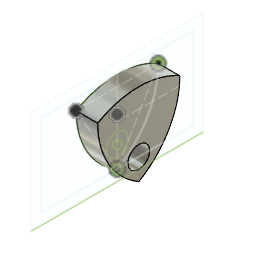
final_oarecum (Autodesk Fusion 360 archive; units mm, degrees)
design "ruleaux"
part number: 2026-06-01-21-01-21-214
Autodesk Fusion 360 part; units mm, degrees
sketch "Excentric Triunghiular Ruleaux + Frame-ul cadrului culisant" plane through (0, 0, 0) normal (1, 0, 0) x (0, 1, 0)
  line L0 (-9.5, 5.4848) -> (0, -10.9697) construction
  line L1 (0, -10.9697) -> (9.5, 5.4848) construction
  line L2 (9.5, 5.4848) -> (-9.5, 5.4848) construction
  arc A0 (0, -10.9697) -> (9.5, 5.4848) centre (-9.5, 5.4848) ccw
  arc A1 (-9.5, 5.4848) -> (0, -10.9697) centre (9.5, 5.4848) ccw
  arc A2 (9.5, 5.4848) -> (-9.5, 5.4848) centre (0, -10.9697) ccw
  circle A3 centre (0, -6) radius 2.5
  line L3 (-17.5, 8.0303) -> (17.5, 8.0303)
  line L4 (17.5, 8.0303) -> (17.5, -10.9697)
  line L5 (17.5, -10.9697) -> (-17.5, -10.9697)
  line L6 (-17.5, -10.9697) -> (-17.5, 8.0303)
  line L7 (0, 8.0303) -> (0, -10.9697) construction
  line L8 (20, -13.4697) -> (-20, -13.4697)
  line L9 (-20, -13.4697) -> (-20, 10.5303)
  line L10 (-20, 10.5303) -> (20, 10.5303)
  line L11 (20, 10.5303) -> (20, -13.4697)
  line L12 (17.5, -1.4697) -> (0, -1.4697) construction
  dimension "d4" = 19
  dimension "d5" = 5
  dimension "d6" = 35
  dimension "d7" = 19
  dimension "d8" = 6
  dimension "d9" = 17.5
  dimension "d10" = -2.5
  constraint coincident L0.start L2.end
  constraint coincident L0.end L1.start
  constraint coincident L0.start A2
  constraint coincident L1.end L2.start
  constraint coincident L0.end A1
  constraint horizontal L3
  constraint vertical L4
  constraint horizontal L5
  constraint vertical L6
  constraint midpoint A2 L7.start
  constraint perpendicular L5 L7
  constraint midpoint L4 L12.start
  constraint midpoint L7 L12.end
  measures "d4" distance of L0.start L1.end
  measures "d5" diameter of A3
  measures "d6" distance of L3.start L3.end
  measures "d7" distance of L3.start L5.end
  measures "d8" distance of origin A3.centre
  measures "d9" distance of L4 L7
extrude "Extrude1" add sketch "Excentric Triunghiular Ruleaux + Frame-ul cadrului culisant" along normal blind 5 contours A0 A1 A2
equation "d9 = ( 35 / 2 ) * 1 mm"
equation "d17 = ( 38 / 2 ) * 1 mm"
named bodies: "Excentric Triunghiular Ruleaux"

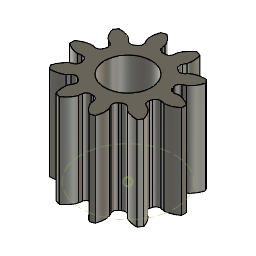
design "gear mic"
part number: 2026-06-01-17-47-26-334
Autodesk Fusion 360 part; units mm, degrees
sketch "Base Circle" plane through (0, 0, 0) normal (0, 0, 1) x (1, 0, 0)
  circle A0 centre (0, 0) radius 3.843
  circle A1 centre (0, 0) radius 2.5
extrude "Extrude3" add sketch "Base Circle" along normal blind 10
sketch "Gear Tooth" plane through (0, 0, 0) normal (0, 0, 1) x (1, 0, 0)
  spline S0 degree 5 poles (4.6331, -0.7809) (4.6369, -0.7816) (4.6445, -0.7827) (4.6559, -0.784) (4.6712, -0.7851) (4.6904, -0.7854) (4.7097, -0.7849) (4.7291, -0.784) (4.7485, -0.7829) (4.7679, -0.7816) (4.7874, -0.7801) (4.8069, -0.7783) (4.8264, -0.7763) (4.8459, -0.7739) (4.8655, -0.7711) (4.8851, -0.768) (4.9048, -0.7646) (4.9244, -0.761) (4.9441, -0.7571) (4.9637, -0.753) (4.9834, -0.7488) (5.0031, -0.7443) (5.0228, -0.7395) (5.0425, -0.7346) (5.0622, -0.7294) (5.0819, -0.7239) (5.1017, -0.7183) (5.1214, -0.7124) (5.1411, -0.7064) (5.1608, -0.7001) (5.1806, -0.6937) (5.2003, -0.6871) (5.22, -0.6802) (5.2397, -0.6732) (5.2594, -0.666) (5.2791, -0.6586) (5.2988, -0.651) (5.3185, -0.6432) (5.3381, -0.6352) (5.3578, -0.6271) (5.3774, -0.6187) (5.3971, -0.6102) (5.4167, -0.6015) (5.4363, -0.5927) (5.4559, -0.5836) (5.4754, -0.5744) (5.495, -0.565) (5.5145, -0.5555) (5.534, -0.5457) (5.5535, -0.5359) (5.573, -0.5258) (5.5924, -0.5156) (5.6119, -0.5052) (5.6313, -0.4946) (5.6506, -0.4839) (5.67, -0.473) (5.6893, -0.4619) (5.7086, -0.4507) (5.7279, -0.4394) (5.7471, -0.4278) (5.7663, -0.4161) (5.7855, -0.4043) (5.8047, -0.3923) (5.8238, -0.3801) (5.8428, -0.3678) (5.8619, -0.3554) (5.8809, -0.3427) (5.8999, -0.33) (5.9188, -0.317) (5.9377, -0.304) (5.9566, -0.2907) (5.9717, -0.28) (5.9829, -0.2719) (5.9904, -0.2665) (5.9942, -0.2638) knots 0 0 0 0 0 0 0.01428571 0.02857143 0.04285714 0.05714286 0.07142857 0.08571429 0.1 0.11428571 0.12857143 0.14285714 0.15714286 0.17142857 0.18571429 0.2 0.21428571 0.22857143 0.24285714 0.25714286 0.27142857 0.28571429 0.3 0.31428571 0.32857143 0.34285714 0.35714286 0.37142857 0.38571429 0.4 0.41428571 0.42857143 0.44285714 0.45714286 0.47142857 0.48571429 0.5 0.51428571 0.52857143 0.54285714 0.55714286 0.57142857 0.58571429 0.6 0.61428571 0.62857143 0.64285714 0.65714286 0.67142857 0.68571429 0.7 0.71428571 0.72857143 0.74285714 0.75714286 0.77142857 0.78571429 0.8 0.81428571 0.82857143 0.84285714 0.85714286 0.87142857 0.88571429 0.9 0.91428571 0.92857143 0.94285714 0.95714286 0.97142857 0.98571429 1 1 1 1 1 1
  spline S1 degree 5 poles (4.6331, 0.7809) (4.6369, 0.7816) (4.6445, 0.7827) (4.6559, 0.784) (4.6712, 0.7851) (4.6904, 0.7854) (4.7097, 0.7849) (4.7291, 0.784) (4.7485, 0.7829) (4.7679, 0.7816) (4.7874, 0.7801) (4.8069, 0.7783) (4.8264, 0.7763) (4.8459, 0.7739) (4.8655, 0.7711) (4.8851, 0.768) (4.9048, 0.7646) (4.9244, 0.761) (4.9441, 0.7571) (4.9637, 0.753) (4.9834, 0.7488) (5.0031, 0.7443) (5.0228, 0.7395) (5.0425, 0.7346) (5.0622, 0.7294) (5.0819, 0.7239) (5.1017, 0.7183) (5.1214, 0.7124) (5.1411, 0.7064) (5.1608, 0.7001) (5.1806, 0.6937) (5.2003, 0.6871) (5.22, 0.6802) (5.2397, 0.6732) (5.2594, 0.666) (5.2791, 0.6586) (5.2988, 0.651) (5.3185, 0.6432) (5.3381, 0.6352) (5.3578, 0.6271) (5.3774, 0.6187) (5.3971, 0.6102) (5.4167, 0.6015) (5.4363, 0.5927) (5.4559, 0.5836) (5.4754, 0.5744) (5.495, 0.565) (5.5145, 0.5555) (5.534, 0.5457) (5.5535, 0.5359) (5.573, 0.5258) (5.5924, 0.5156) (5.6119, 0.5052) (5.6313, 0.4946) (5.6506, 0.4839) (5.67, 0.473) (5.6893, 0.4619) (5.7086, 0.4507) (5.7279, 0.4394) (5.7471, 0.4278) (5.7663, 0.4161) (5.7855, 0.4043) (5.8047, 0.3923) (5.8238, 0.3801) (5.8428, 0.3678) (5.8619, 0.3554) (5.8809, 0.3427) (5.8999, 0.33) (5.9188, 0.317) (5.9377, 0.304) (5.9566, 0.2907) (5.9717, 0.28) (5.9829, 0.2719) (5.9904, 0.2665) (5.9942, 0.2638) knots 0 0 0 0 0 0 0.01428571 0.02857143 0.04285714 0.05714286 0.07142857 0.08571429 0.1 0.11428571 0.12857143 0.14285714 0.15714286 0.17142857 0.18571429 0.2 0.21428571 0.22857143 0.24285714 0.25714286 0.27142857 0.28571429 0.3 0.31428571 0.32857143 0.34285714 0.35714286 0.37142857 0.38571429 0.4 0.41428571 0.42857143 0.44285714 0.45714286 0.47142857 0.48571429 0.5 0.51428571 0.52857143 0.54285714 0.55714286 0.57142857 0.58571429 0.6 0.61428571 0.62857143 0.64285714 0.65714286 0.67142857 0.68571429 0.7 0.71428571 0.72857143 0.74285714 0.75714286 0.77142857 0.78571429 0.8 0.81428571 0.82857143 0.84285714 0.85714286 0.87142857 0.88571429 0.9 0.91428571 0.92857143 0.94285714 0.95714286 0.97142857 0.98571429 1 1 1 1 1 1
  arc A0 (5.9942, -0.2638) -> (5.9942, 0.2638) centre (0, 0) ccw
  line L0 (3.7797, -0.6371) -> (4.6331, -0.7809)
  line L1 (3.7797, 0.6371) -> (4.6331, 0.7809)
  line L2 (3.7797, -0.6371) -> (3.7797, 0.6371)
  point P0 (4.7268, -0.7841)
  point P1 (4.8223, -0.7767)
  point P2 (4.9187, -0.762)
  point P3 (5.0159, -0.7412)
  point P4 (5.1136, -0.7147)
  point P5 (5.2117, -0.6831)
  point P6 (5.31, -0.6465)
  point P7 (5.4084, -0.6052)
  point P8 (5.5068, -0.5592)
  point P9 (5.6051, -0.5088)
  point P10 (5.7031, -0.4539)
  point P11 (5.8006, -0.3948)
  point P12 (5.8977, -0.3314)
  point P13 (4.7268, 0.7841)
  point P14 (4.8223, 0.7767)
  point P15 (4.9187, 0.762)
  point P16 (5.0159, 0.7412)
  point P17 (5.1136, 0.7147)
  point P18 (5.2117, 0.6831)
  point P19 (5.31, 0.6465)
  point P20 (5.4084, 0.6052)
  point P21 (5.5068, 0.5592)
  point P22 (5.6051, 0.5088)
  point P23 (5.7031, 0.4539)
  point P24 (5.8006, 0.3948)
  point P25 (5.8977, 0.3314)
extrude "Extrude4" add sketch "Gear Tooth" along normal blind 10
fillet "Fillet2" radius 0.5 2 edges at (3.7895, -0.6387, 5) (3.7895, 0.6387, 5)
pattern_circular "C-Pattern2" count 10 over 360 about axis through (0, 0, 0) along (0, 0, 1) of "Extrude4", "Fillet2"
sketch "Diametrial Pitch Circle" plane through (0, 0, 0) normal (0, 0, 1) x (1, 0, 0)
  circle A0 centre (0, 0) radius 5 construction
named bodies: "Spur Gear (10 teeth)"

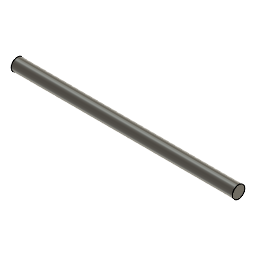
design "ax"
part number: 2026-06-02-10-52-54-374
Autodesk Fusion 360 part; units mm, degrees
sketch "Ax" plane through (0, 0, 0) normal (1, 0, 0) x (0, 1, 0)
  circle A0 centre (0, 0) radius 2.25
  dimension "d1" = 4.5
  constraint coincident A0.centre origin
  measures "d1" diameter of A0
extrude "Extrude1" add sketch "Ax" along normal blind 80
named bodies: "Ax"

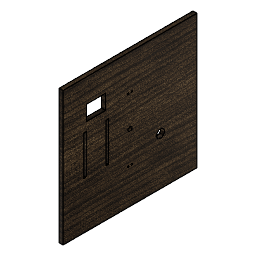
design "plate"
part number: 2026-06-01-11-50-28-145
Autodesk Fusion 360 part; units mm, degrees
sketch "Plate" plane through (0, 0, 0) normal (1, 0, 0) x (0, 1, 0)
  line L0 (95, 95) -> (-95, 95)
  line L1 (-95, 95) -> (-95, -95)
  line L2 (-95, -95) -> (95, -95)
  line L3 (95, -95) -> (95, 95)
  line L4 (95, 95) -> (-95, -95) construction
  line L5 (-95, 95) -> (95, -95) construction
  line L6 (90, -90) -> (90, 90)
  line L7 (90, 90) -> (-90, 90)
  line L8 (-90, 90) -> (-90, -90)
  line L9 (-90, -90) -> (90, -90)
  line L10 (85, -85) -> (85, 85)
  line L11 (85, 85) -> (-85, 85)
  line L12 (-85, 85) -> (-85, -85)
  line L13 (-85, -85) -> (85, -85)
  circle A0 centre (0, 0) radius 2.5
  line L14 (-55, 55) -> (-31, 55)
  line L15 (-31, 55) -> (-31, 36)
  line L16 (-31, 36) -> (-55, 36)
  line L17 (-55, 36) -> (-55, 55)
  line L18 (-57.0845, 85) -> (-57.0845, -85) construction
  line L19 (-28.9155, 85) -> (-28.9155, -85) construction
  line L20 (-55.5845, 25) -> (-58.5845, 25)
  line L21 (-58.5845, 25) -> (-58.5845, -25)
  line L22 (-58.5845, -25) -> (-55.5845, -25)
  line L23 (-55.5845, -25) -> (-55.5845, 25)
  line L24 (-85, 0) -> (85, 0) construction
  line L25 (-30.3955, 25) -> (-30.3955, -25)
  line L26 (-27.3955, -25) -> (-27.3955, 25)
  line L27 (-30.3955, -25) -> (-27.3955, -25)
  line L28 (-27.3955, 25) -> (-30.3955, 25)
  line L29 (0, 85) -> (0, -85) construction
  circle A1 centre (38.833, -24.365) radius 5
  circle A2 centre (-2.3875, 40) radius 1
  circle A3 centre (2.3875, 40) radius 1
  circle A4 centre (-2.3875, -40) radius 1
  circle A5 centre (2.3875, -40) radius 1
  line L30 (-43, 0) -> (-43, -9.5) construction
  line L31 (-43, 0) -> (-43, 9.5) construction
  dimension "d1" = 190
  dimension "d2" = 190
  dimension "d3" = -5
  dimension "d4" = -5
  dimension "d5" = 5
  dimension "d6" = 24
  dimension "d7" = 19
  dimension "d8" = 30
  dimension "d9" = 30
  dimension "d10" = 28.169
  dimension "d11" = 2.0845
  dimension "d12" = 50
  dimension "d13" = 3
  dimension "d14" = 1.5
  dimension "d15" = 25
  dimension "d16" = 50
  dimension "d17" = 3
  dimension "d18" = 25.189
  dimension "d19" = 25
  dimension "d29" = 10
  dimension "d30" = 24.365
  dimension "d31" = 38.833
  dimension "d35" = 2
  dimension "d36" = 2
  dimension "d37" = 4.775
  dimension "d38" = 40
  dimension "d39" = 2.3875
  dimension "d40" = 40
  dimension "d41" = 9.5
  dimension "d42" = 9.5
  constraint horizontal L0
  constraint perpendicular L0 L1
  constraint parallel L0 L2
  constraint parallel L1 L3
  constraint coincident L4 A0.centre
  constraint coincident L5 A0.centre
  constraint coincident A0.centre origin
  constraint horizontal L14
  constraint vertical L15
  constraint horizontal L16
  constraint vertical L17
  constraint coincident L11 L18.start
  constraint coincident L13 L18.end
  constraint perpendicular L13 L18
  constraint coincident L11 L19.start
  constraint coincident L13 L19.end
  constraint perpendicular L13 L19
  constraint horizontal L20
  constraint vertical L21
  constraint horizontal L22
  constraint vertical L23
  constraint midpoint L12 L24.start
  constraint midpoint L10 L24.end
  constraint horizontal L28
  constraint vertical L25
  constraint horizontal L27
  constraint vertical L26
  constraint midpoint L11 L29.start
  constraint midpoint L13 L29.end
  constraint symmetric L24 A2 A4
  constraint symmetric L24 A3 A5
  constraint coincident L24 L30.start
  constraint perpendicular L24 L30
  constraint perpendicular L24 L31
  measures "d1" distance of L1.end L2.end
  measures "d2" distance of L0.end L1.end
  measures "d5" diameter of A0
  measures "d6" distance of L14.start L14.end
  measures "d7" distance of L14.start L16.end
  measures "d8" distance of L12 L17
  measures "d9" distance of L11 L14
  measures "d10" distance of L18 L19
  measures "d11" distance of L15 L19
  measures "d12" distance of L20.end L21.end
  measures "d13" distance of L21 L23
  measures "d14" distance of L18 L23
  measures "d15" distance of L20 L24
  measures "d16" distance of L25.end L25.start
  measures "d17" distance of L25 L26
  measures "d18" distance of L23 L25
  measures "d19" distance of L24 L28
  measures "d29" diameter of A1
  measures "d30" distance of L24 A1.centre
  measures "d31" distance of L29 A1.centre
  measures "d35" diameter of A2
  measures "d36" diameter of A3
  measures "d37" horizontal distance of A2.centre A3.centre
  measures "d38" distance of L24 A2.centre
  measures "d39" distance of L29 A2.centre
  measures "d40" distance of L24 A3.centre
  measures "d41" distance of L30.start L30.end
  measures "d42" distance of L30.start L31.end
extrude "Extrude1" add sketch "Plate" along normal mid plane 5 contours L10 L11 L12 L13
equation "d2 = d1"
equation "d8 = ( 30 * d1 / 190 mm ) * 1 mm"
equation "d9 = ( 30 * d1 / 190 mm ) * 1 mm"
equation "d11 = ( ( 28.169 - 24 ) / 2 ) * 1 mm"
equation "d16 = d12"
equation "d17 = d13"
equation "d19 = d15"
equation "d39 = ( 4.775 / 2 ) * 1 mm"
named bodies: "plate"

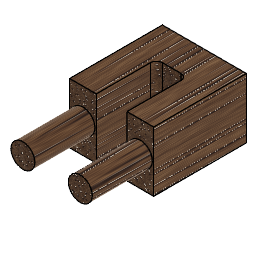
design "Prindere Cadru"
part number: 2026-06-01-23-22-02-267
Autodesk Fusion 360 part; units mm, degrees
sketch "baza" plane through (0, 0, 0) normal (0, 0, 1) x (1, 0, 0)
  line L0 (1.275, 1.275) -> (-1.275, 1.275)
  line L1 (-1.275, 1.275) -> (-1.275, -1.275)
  line L2 (-1.275, -1.275) -> (1.275, -1.275)
  line L3 (1.275, -1.275) -> (1.275, 1.275)
  line L4 (1.275, 1.275) -> (-1.275, -1.275) construction
  line L5 (-1.275, 1.275) -> (1.275, -1.275) construction
  line L6 (3.5, 0) -> (3.5, -1.275)
  line L7 (-3.5, -1.275) -> (-3.5, 0)
  line L8 (-1.275, -1.275) -> (-3.5, -1.275)
  line L9 (1.275, -1.275) -> (3.5, -1.275)
  line L10 (3.5, 0) -> (3.5, 4)
  line L11 (3.5, 4) -> (-3.5, 4)
  line L12 (-3.5, 4) -> (-3.5, 0)
  line L13 (-1.275, -1.275) -> (-1.275, -3.725)
  line L14 (1.275, -1.275) -> (1.275, -3.725)
  line L15 (1.275, -3.725) -> (3.5, -3.725)
  line L16 (3.5, -3.725) -> (3.5, -1.275)
  line L17 (-3.5, -1.275) -> (-3.5, -3.725)
  line L18 (-3.5, -3.725) -> (-1.275, -3.725)
  line L19 (-1.275, 0.775) -> (1.275, 0.775)
  dimension "d1" = 2.55
  dimension "d4" = 7
  dimension "d11" = 7
  dimension "d12" = 4
  dimension "d16" = 1.275
  dimension "d17" = 2.45
  dimension "d18" = 0.5
  constraint horizontal L0
  constraint perpendicular L0 L1
  constraint parallel L0 L2
  constraint parallel L1 L3
  constraint coincident L4 origin
  constraint coincident L5 origin
  constraint vertical L6
  constraint vertical L7
  constraint perpendicular L7 L8
  constraint perpendicular L6 L9
  constraint vertical L10
  constraint horizontal L11
  constraint vertical L12
  constraint perpendicular L2 L13
  constraint perpendicular L2 L14
  constraint perpendicular L6 L15
  constraint perpendicular L9 L16
  constraint perpendicular L8 L17
  constraint perpendicular L13 L18
  constraint coincident L1 L19.start
  constraint coincident L3 L19.end
  constraint perpendicular L3 L19
  measures "d1" distance of L1.end L2.end
  measures "d4" distance of L7.end L6.start
  measures "d11" distance of L7.end L6.start
  measures "d12" distance of L7.end L11.end
  measures "d16" distance of L2 origin
  measures "d17" distance of L1.end L13.end
  measures "d18" distance of L0 L19
extrude "Extrude1" add sketch "baza" along normal blind 5 contours L0 L1 L3 L6 L7 L8 L9 L10 L11 L12 | L9 L14 L15 L16 | L8 L13 L17 L18
sketch "dinti" plane through (0, -3.725, 0) normal (0, -1, 0) x (1, 0, 0)
  line L0 (-3.5, 0) -> (-1.275, 0)
  line L1 (-1.275, 0) -> (-1.275, 5)
  line L2 (-1.275, 5) -> (-3.5, 5)
  line L3 (-3.5, 5) -> (-3.5, 0)
  line L4 (-2.3875, 5) -> (-2.3875, 0) construction
  circle A0 centre (-2.3875, 2.5) radius 1
  line L5 (-1.275, 0) -> (1.275, 0) construction
  line L6 (1.275, 0) -> (1.275, 5) construction
  line L7 (1.275, 5) -> (-1.275, 5) construction
  line L8 (-1.275, 5) -> (-1.275, 0) construction
  line L9 (0, 5) -> (0, 0) construction
  circle A1 centre (2.3875, 2.5) radius 1
  line L10 (-3.5, 0) -> (-1.275, 0)
  line L11 (-1.275, 0) -> (-1.275, 5)
  line L12 (-1.275, 5) -> (-3.5, 5)
  line L13 (-3.5, 5) -> (-3.5, 0)
  dimension "d8" = 2
  constraint midpoint L2 L4.start
  constraint midpoint L0 L4.end
  constraint midpoint L4 A0.centre
  constraint midpoint L7 L9.start
  constraint coincident L9.end origin
  constraint symmetric A0 L9 A1
  measures "d8" diameter of A0
extrude "Extrude2" add sketch "dinti" along normal blind 5 contours A0 | A1
fillet "Fillet1" radius 0.5 2 edges at (1.275, 1.275, 2.5) (-1.275, 1.275, 2.5)
equation "d17 = 3.725 mm - 1.275 mm"
named bodies: "Prindere"

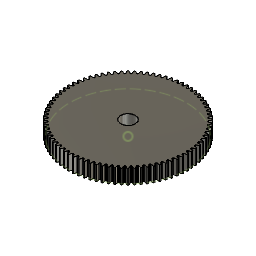
design "gear mare"
part number: 2026-06-01-18-08-30-536
Autodesk Fusion 360 part; units mm, degrees
sketch "Base Circle" plane through (0, 0, 0) normal (0, 0, 1) x (1, 0, 0)
  circle A0 centre (0, 0) radius 38.843
  circle A1 centre (0, 0) radius 5
extrude "Extrude1" add sketch "Base Circle" along normal blind 10
sketch "Gear Tooth" plane through (0, 0, 0) normal (0, 0, 1) x (1, 0, 0)
  spline S0 degree 5 poles (37.5661, -1.2745) (37.576, -1.2745) (37.5958, -1.2743) (37.6254, -1.2737) (37.665, -1.2726) (37.7145, -1.2705) (37.764, -1.2677) (37.8134, -1.2641) (37.8629, -1.26) (37.9124, -1.2552) (37.9618, -1.2498) (38.0113, -1.244) (38.0608, -1.2377) (38.1102, -1.2311) (38.1597, -1.2241) (38.2091, -1.2167) (38.2585, -1.209) (38.3079, -1.201) (38.3573, -1.1926) (38.4067, -1.1838) (38.4561, -1.1748) (38.5054, -1.1654) (38.5548, -1.1557) (38.6041, -1.1457) (38.6534, -1.1355) (38.7027, -1.1249) (38.752, -1.1141) (38.8013, -1.103) (38.8506, -1.0917) (38.8998, -1.0801) (38.949, -1.0682) (38.9983, -1.0561) (39.0474, -1.0437) (39.0966, -1.0311) (39.1458, -1.0182) (39.1949, -1.0051) (39.2441, -0.9918) (39.2932, -0.9782) (39.3422, -0.9644) (39.3913, -0.9504) (39.4404, -0.9361) (39.4894, -0.9217) (39.5384, -0.907) (39.5874, -0.8921) (39.6364, -0.8769) (39.6853, -0.8616) (39.7342, -0.8461) (39.7831, -0.8303) (39.832, -0.8143) (39.8809, -0.7982) (39.9297, -0.7818) (39.9786, -0.7653) (40.0274, -0.7485) (40.0761, -0.7315) (40.1249, -0.7144) (40.1736, -0.697) (40.2223, -0.6795) (40.271, -0.6618) (40.3197, -0.6439) (40.3683, -0.6258) (40.4169, -0.6075) (40.4655, -0.589) (40.5141, -0.5703) (40.5626, -0.5515) (40.6111, -0.5325) (40.6596, -0.5133) (40.7081, -0.4939) (40.7565, -0.4743) (40.8049, -0.4546) (40.8533, -0.4347) (40.9017, -0.4146) (40.9403, -0.3984) (40.9693, -0.3861) (40.9886, -0.3779) (40.9983, -0.3738) knots 0 0 0 0 0 0 0.01428571 0.02857143 0.04285714 0.05714286 0.07142857 0.08571429 0.1 0.11428571 0.12857143 0.14285714 0.15714286 0.17142857 0.18571429 0.2 0.21428571 0.22857143 0.24285714 0.25714286 0.27142857 0.28571429 0.3 0.31428571 0.32857143 0.34285714 0.35714286 0.37142857 0.38571429 0.4 0.41428571 0.42857143 0.44285714 0.45714286 0.47142857 0.48571429 0.5 0.51428571 0.52857143 0.54285714 0.55714286 0.57142857 0.58571429 0.6 0.61428571 0.62857143 0.64285714 0.65714286 0.67142857 0.68571429 0.7 0.71428571 0.72857143 0.74285714 0.75714286 0.77142857 0.78571429 0.8 0.81428571 0.82857143 0.84285714 0.85714286 0.87142857 0.88571429 0.9 0.91428571 0.92857143 0.94285714 0.95714286 0.97142857 0.98571429 1 1 1 1 1 1
  spline S1 degree 5 poles (37.5661, 1.2745) (37.576, 1.2745) (37.5958, 1.2743) (37.6254, 1.2737) (37.665, 1.2726) (37.7145, 1.2705) (37.764, 1.2677) (37.8134, 1.2641) (37.8629, 1.26) (37.9124, 1.2552) (37.9618, 1.2498) (38.0113, 1.244) (38.0608, 1.2377) (38.1102, 1.2311) (38.1597, 1.2241) (38.2091, 1.2167) (38.2585, 1.209) (38.3079, 1.201) (38.3573, 1.1926) (38.4067, 1.1838) (38.4561, 1.1748) (38.5054, 1.1654) (38.5548, 1.1557) (38.6041, 1.1457) (38.6534, 1.1355) (38.7027, 1.1249) (38.752, 1.1141) (38.8013, 1.103) (38.8506, 1.0917) (38.8998, 1.0801) (38.949, 1.0682) (38.9983, 1.0561) (39.0474, 1.0437) (39.0966, 1.0311) (39.1458, 1.0182) (39.1949, 1.0051) (39.2441, 0.9918) (39.2932, 0.9782) (39.3422, 0.9644) (39.3913, 0.9504) (39.4404, 0.9361) (39.4894, 0.9217) (39.5384, 0.907) (39.5874, 0.8921) (39.6364, 0.8769) (39.6853, 0.8616) (39.7342, 0.8461) (39.7831, 0.8303) (39.832, 0.8143) (39.8809, 0.7982) (39.9297, 0.7818) (39.9786, 0.7653) (40.0274, 0.7485) (40.0761, 0.7315) (40.1249, 0.7144) (40.1736, 0.697) (40.2223, 0.6795) (40.271, 0.6618) (40.3197, 0.6439) (40.3683, 0.6258) (40.4169, 0.6075) (40.4655, 0.589) (40.5141, 0.5703) (40.5626, 0.5515) (40.6111, 0.5325) (40.6596, 0.5133) (40.7081, 0.4939) (40.7565, 0.4743) (40.8049, 0.4546) (40.8533, 0.4347) (40.9017, 0.4146) (40.9403, 0.3984) (40.9693, 0.3861) (40.9886, 0.3779) (40.9983, 0.3738) knots 0 0 0 0 0 0 0.01428571 0.02857143 0.04285714 0.05714286 0.07142857 0.08571429 0.1 0.11428571 0.12857143 0.14285714 0.15714286 0.17142857 0.18571429 0.2 0.21428571 0.22857143 0.24285714 0.25714286 0.27142857 0.28571429 0.3 0.31428571 0.32857143 0.34285714 0.35714286 0.37142857 0.38571429 0.4 0.41428571 0.42857143 0.44285714 0.45714286 0.47142857 0.48571429 0.5 0.51428571 0.52857143 0.54285714 0.55714286 0.57142857 0.58571429 0.6 0.61428571 0.62857143 0.64285714 0.65714286 0.67142857 0.68571429 0.7 0.71428571 0.72857143 0.74285714 0.75714286 0.77142857 0.78571429 0.8 0.81428571 0.82857143 0.84285714 0.85714286 0.87142857 0.88571429 0.9 0.91428571 0.92857143 0.94285714 0.95714286 0.97142857 0.98571429 1 1 1 1 1 1
  arc A0 (40.9983, -0.3738) -> (40.9983, 0.3738) centre (0, 0) ccw
  line L0 (37.5661, 1.2745) -> (37.5661, -1.2745)
  point P0 (37.8103, -1.2642)
  point P1 (38.055, -1.2384)
  point P2 (38.3, -1.2022)
  point P3 (38.5453, -1.1575)
  point P4 (38.7906, -1.1054)
  point P5 (39.0361, -1.0465)
  point P6 (39.2816, -0.9814)
  point P7 (39.5271, -0.9103)
  point P8 (39.7726, -0.8337)
  point P9 (40.018, -0.7517)
  point P10 (40.2633, -0.6645)
  point P11 (40.5085, -0.5724)
  point P12 (40.7535, -0.4755)
  point P13 (37.8103, 1.2642)
  point P14 (38.055, 1.2384)
  point P15 (38.3, 1.2022)
  point P16 (38.5453, 1.1575)
  point P17 (38.7906, 1.1054)
  point P18 (39.0361, 1.0465)
  point P19 (39.2816, 0.9814)
  point P20 (39.5271, 0.9103)
  point P21 (39.7726, 0.8337)
  point P22 (40.018, 0.7517)
  point P23 (40.2633, 0.6645)
  point P24 (40.5085, 0.5724)
  point P25 (40.7535, 0.4755)
extrude "Extrude2" add sketch "Gear Tooth" along normal blind 10
fillet "Fillet1" radius 0.5 2 edges at (38.8275, 1.097, 5) (38.8275, -1.097, 5)
pattern_circular "C-Pattern1" count 80 over 360 about axis through (0, 0, 0) along (0, 0, 1) of "Extrude2", "Fillet1"
sketch "Diametrial Pitch Circle" plane through (0, 0, 0) normal (0, 0, 1) x (1, 0, 0)
  circle A0 centre (0, 0) radius 40 construction
named bodies: "Spur Gear (80 teeth)"

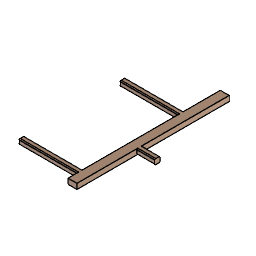
design "Furcă"
part number: 2026-06-02-07-13-39-938
Autodesk Fusion 360 part; units mm, degrees
sketch "Sketch1" plane through (0, 0, 0) normal (0, 0, 1) x (1, 0, 0)
  line L0 (-1.25, 17.5) -> (1.25, 17.5)
  line L1 (1.25, 17.5) -> (1.25, -17.5)
  line L2 (1.25, -17.5) -> (-1.25, -17.5)
  line L3 (-1.25, -17.5) -> (-1.25, 17.5)
  line L4 (-1.25, 17.5) -> (1.25, -17.5) construction
  line L5 (1.25, 17.5) -> (-1.25, -17.5) construction
  line L6 (0, 0) -> (0, -14.0845) construction
  line L7 (-1.25, -14.8345) -> (-17.75, -14.8345)
  line L8 (-17.75, -14.8345) -> (-17.75, -13.3345)
  line L9 (-17.75, -13.3345) -> (-1.25, -13.3345)
  line L10 (1.25, -0.775) -> (6.25, -0.775)
  line L11 (6.25, -0.775) -> (6.25, 0.725)
  line L12 (6.25, 0.725) -> (1.25, 0.725)
  line L13 (0, -14.0845) -> (-16.5, -14.0845) construction
  line L14 (0, 0) -> (-10.5, 0) construction
  line L15 (-17.75, 13.3345) -> (-1.25, 13.3345)
  line L16 (-1.25, 14.8345) -> (-17.75, 14.8345)
  line L17 (-17.75, 13.3345) -> (-17.75, 14.8345)
  line L18 (-1.25, 17.5) -> (-1.25, 25)
  line L19 (1.25, 17.5) -> (1.25, 25)
  line L20 (1.25, 25) -> (-1.25, 25)
  dimension "d1" = 35
  dimension "d2" = 14.0845
  dimension "d3" = 0.75
  dimension "d4" = 1.5
  dimension "d5" = 16.5
  dimension "d6" = 1.5
  dimension "d7" = 0.775
  dimension "d8" = 5
  dimension "d9" = 2.5
  dimension "d10" = 16.5
  dimension "d19" = 7.5
  dimension "d20" = 7.5
  constraint horizontal L0
  constraint perpendicular L0 L1
  constraint parallel L0 L2
  constraint parallel L1 L3
  constraint coincident L4 L6.start
  constraint coincident L5 L6.start
  constraint coincident L6.start L14.start
  constraint parallel L3 L6
  constraint coincident L3 L7.start
  constraint perpendicular L3 L7
  constraint perpendicular L7 L8
  constraint coincident L3 L9.end
  constraint perpendicular L3 L9
  constraint coincident L1 L10.start
  constraint perpendicular L1 L10
  constraint perpendicular L10 L11
  constraint coincident L1 L12.end
  constraint perpendicular L1 L12
  constraint perpendicular L6 L13
  constraint perpendicular L6 L14
  constraint symmetric L7.start L14 L16.start
  constraint symmetric L7.end L14 L16.end
  constraint symmetric L8.end L14 L15.start
  constraint symmetric L9.end L14 L15.end
  constraint perpendicular L0 L18
  constraint perpendicular L0 L19
  measures "d1" distance of L0.end L1.end
  measures "d2" distance of L6.start L6.end
  measures "d3" distance of L6.end L7
  measures "d4" distance of L7.end L8.end
  measures "d5" distance of L7.start L7.end
  measures "d6" distance of L10.end L11.end
  measures "d7" distance of L6.start L10
  measures "d8" distance of L1 L11
  measures "d9" distance of L1.end L2.end
  measures "d10" distance of L6.end L13.end
  measures "d19" distance of L0.start L18.end
  measures "d20" distance of L0.end L19.end
extrude "Extrude1" add sketch "Sketch1" along normal blind 1.5
fillet "Fillet1" radius 0.25 4 edges at (3.75, -0.775, 1.5) (3.75, -0.775, 0) (3.75, 0.725, 0) (3.75, 0.725, 1.5)
fillet "Fillet2" radius 0.25 4 edges at (-9.5, -14.8345, 1.5) (-9.5, -13.3345, 1.5) (-9.5, -13.3345, 0) (-9.5, -14.8345, 0)
fillet "Fillet3" radius 0.25 4 edges at (-9.5, 14.8345, 1.5) (-9.5, 13.3345, 1.5) (-9.5, 14.8345, 0) (-9.5, 13.3345, 0)
fillet "Fillet4" radius 0.25 16 edges at (-17.75, -14.8345, 0.75) (-17.75, -14.7613, 0.0732) (-17.75, -14.0845, 0) (-17.75, -13.4077, 0.0732) (-17.75, -13.3345, 0.75) (-17.75, -13.4077, 1.4268) (-17.75, -14.0845, 1.5) (-17.75, -14.7613, 1.4268) (-17.75, 13.3345, 0.75) (-17.75, 13.4077, 0.0732) (-17.75, 14.0845, 0) (-17.75, 14.7613, 0.0732) (-17.75, 14.8345, 0.75) (-17.75, 14.7613, 1.4268) (-17.75, 14.0845, 1.5) (-17.75, 13.4077, 1.4268)
equation "d2 = ( 28.169 / 2 ) * 1 mm"
equation "d3 = ( 1.5 / 2 ) * 1 mm"
equation "d7 = ( 1.55 / 2 ) * 1 mm"
named bodies: "furca"

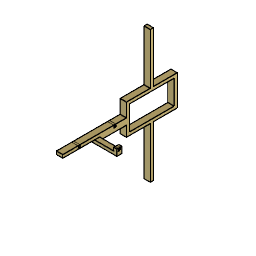
design "Cadru Culisant"
part number: 2026-06-01-23-46-25-790
Autodesk Fusion 360 part; units mm, degrees
sketch "cadru" plane through (0, 0, 0) normal (1, 0, 0) x (0, 1, 0)
  line L0 (-20, -13.4697) -> (-20, 10.5303)
  line L1 (-17.5, -10.9697) -> (-17.5, 8.0303)
  line L2 (17.5, -10.9697) -> (-17.5, -10.9697)
  line L3 (20, -13.4697) -> (-20, -13.4697)
  line L4 (17.5, 8.0303) -> (17.5, -10.9697)
  line L5 (20, 10.5303) -> (20, -13.4697)
  line L6 (-20, 10.5303) -> (20, 10.5303)
  line L7 (-17.5, 8.0303) -> (17.5, 8.0303)
  line L8 (-1.25, 10.5303) -> (-1.25, 50.5303)
  line L9 (0, 0) -> (0, 50) construction
  line L10 (1.25, 10.5303) -> (1.25, 50.5303)
  line L11 (-1.25, 50.5303) -> (1.25, 50.5303)
  line L12 (17.5, -1.4697) -> (0, -1.4697) construction
  line L13 (-1.25, -53.4697) -> (1.25, -53.4697)
  line L14 (-1.25, -13.4697) -> (-1.25, -53.4697)
  line L15 (1.25, -13.4697) -> (1.25, -53.4697)
  line L16 (-20, -0.2197) -> (-70, -0.2197)
  line L17 (-70, -0.2197) -> (-70, -2.7197)
  line L18 (-70, -2.7197) -> (-20, -2.7197)
  line L19 (0, -1.4697) -> (-28.916, -1.4697) construction
  line L20 (-28.916, -1.4697) -> (-57.085, -1.4697) construction
  line L21 (-56.31, -0.6947) -> (-57.86, -0.6947)
  line L22 (-57.86, -0.6947) -> (-57.86, -2.2447)
  line L23 (-57.86, -2.2447) -> (-56.31, -2.2447)
  line L24 (-56.31, -2.2447) -> (-56.31, -0.6947)
  line L25 (-56.31, -0.6947) -> (-57.86, -2.2447) construction
  line L26 (-57.86, -0.6947) -> (-56.31, -2.2447) construction
  line L27 (-43.0005, -1.4697) -> (-43.0005, -15) construction
  line L28 (-45.0005, -5.2197) -> (-20, -5.2197)
  line L29 (-45.0005, -5.2197) -> (-45.0005, -0.2197)
  line L30 (-41.0005, -0.2197) -> (-41.0005, -5.2197)
  line L31 (-42.2255, -0.6947) -> (-43.7755, -0.6947)
  line L32 (-43.7755, -0.6947) -> (-43.7755, -2.2447)
  line L33 (-43.7755, -2.2447) -> (-42.2255, -2.2447)
  line L34 (-42.2255, -2.2447) -> (-42.2255, -0.6947)
  line L35 (-42.2255, -0.6947) -> (-43.7755, -2.2447) construction
  line L36 (-43.7755, -0.6947) -> (-42.2255, -2.2447) construction
  line L37 (-28.141, -0.6947) -> (-29.691, -0.6947)
  line L38 (-29.691, -0.6947) -> (-29.691, -2.2447)
  line L39 (-29.691, -2.2447) -> (-28.141, -2.2447)
  line L40 (-28.141, -2.2447) -> (-28.141, -0.6947)
  line L41 (-28.141, -0.6947) -> (-29.691, -2.2447) construction
  line L42 (-29.691, -0.6947) -> (-28.141, -2.2447) construction
  point P0 (-57.085, -1.4697)
  point P1 (-43.0005, -1.4697)
  point P2 (-28.916, -1.4697)
  dimension "d1" = -2.5
  dimension "d2" = 35
  dimension "d3" = 19
  dimension "d4" = 8.0303
  dimension "d5" = 17.5
  dimension "d6" = 40
  dimension "d7" = 1.25
  dimension "d10" = 50
  dimension "d11" = 2.5
  dimension "d12" = 1.25
  dimension "d13" = 28.916
  dimension "d15" = 28.169
  dimension "d16" = 1.55
  dimension "d17" = 1.55
  dimension "d22" = 14.0845
  dimension "d23" = 2.5
  dimension "d24" = 2
  dimension "d25" = 2
  dimension "d26" = 1.55
  dimension "d27" = 1.55
  dimension "d33" = 1.55
  dimension "d34" = 1.55
  dimension "d32" = 0
  constraint horizontal L7
  constraint vertical L4
  constraint horizontal L2
  constraint vertical L1
  constraint coincident L6 L8.start
  constraint perpendicular L6 L8
  constraint coincident L9.start origin
  constraint symmetric L8.start L9 L10.start
  constraint symmetric L8.end L9 L10.end
  constraint midpoint L4 L12.start
  constraint perpendicular L4 L12
  constraint symmetric L8.start L12 L14.start
  constraint symmetric L8.end L12 L13.start
  constraint symmetric L10.start L12 L15.start
  constraint symmetric L10.end L12 L13.end
  constraint coincident L0 L16.start
  constraint perpendicular L0 L16
  constraint perpendicular L16 L17
  constraint coincident L0 L18.end
  constraint perpendicular L0 L18
  constraint perpendicular L0 L19
  constraint parallel L19 L20
  constraint horizontal L21
  constraint perpendicular L21 L22
  constraint parallel L21 L23
  constraint parallel L22 L24
  constraint coincident L25 P0
  constraint coincident L26 P0
  constraint coincident P0 L20.end
  constraint coincident L20 P1
  constraint perpendicular L20 L27
  constraint coincident L0 L28.end
  constraint perpendicular L0 L28
  constraint coincident L16 L29.end
  constraint perpendicular L16 L29
  constraint coincident L16 L30.start
  constraint coincident L28 L30.end
  constraint perpendicular L28 L30
  constraint horizontal L31
  constraint perpendicular L31 L32
  constraint parallel L31 L33
  constraint parallel L32 L34
  constraint coincident L35 P1
  constraint coincident L36 P1
  constraint coincident P1 L27.start
  constraint horizontal L37
  constraint perpendicular L37 L38
  constraint parallel L37 L39
  constraint parallel L38 L40
  constraint coincident L41 P2
  constraint coincident L42 P2
  constraint coincident P2 L19.end
  measures "d2" distance of L4.start L1.end
  measures "d3" distance of L1.end L1.start
  measures "d4" distance of L9.start L7
  measures "d5" distance of L9.start L1
  measures "d6" distance of L8.start L8.end
  measures "d7" distance of L8 L9
  measures "d10" distance of L16.start L16.end
  measures "d11" distance of L16.end L17.end
  measures "d12" distance of L12 L16
  measures "d13" distance of L12.end P2
  measures "d15" distance of P2 P0
  measures "d16" distance of L22.end L23.end
  measures "d17" distance of L21.end L22.end
  measures "d22" distance of P0 L27
  measures "d23" distance of L18 L28
  measures "d24" distance of L27 L29
  measures "d25" distance of L27 L30
  measures "d26" distance of L32.end L33.end
  measures "d27" distance of L31.end L32.end
  measures "d33" distance of L38.end L39.end
  measures "d34" distance of L37.end L38.end
extrude "Extrude1" add sketch "cadru" along normal blind 5 contours L0 L3 L5 L6 | L0 L18 L28 L30 | L3 L13 L14 L15 | L0 L16 L18 L30 | L16 L18 L29 L30 | L16 L17 L18 L29 | L6 L8 L10 L11 | L31 L32 L33 L34
extrude "Extrude2" add sketch "cadru" along normal blind 20 contours L18 L28 L29 L30
extrude "Extrude3" add sketch "cadru" along normal blind 2.5 from surface at 20 contours L18 L28 L29 L30 | L16 L18 L29 L30
equation "d22 = ( 28.169 / 2 ) * 1 mm"
named bodies: "Cadru culisant"

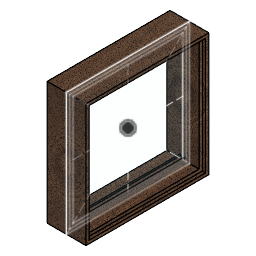
design "cutie"
part number: 2026-06-01-17-19-54-143
Autodesk Fusion 360 part; units mm, degrees
sketch "Sketch1" plane through (0, 0, 0) normal (1, 0, 0) x (0, 1, 0)
  line L0 (90, -90) -> (90, 90)
  line L1 (-95, 95) -> (95, -95) construction
  line L2 (95, 95) -> (-95, 95)
  line L3 (85, 85) -> (-85, 85)
  line L4 (-85, -85) -> (85, -85)
  line L5 (85, -85) -> (85, 85)
  line L6 (-95, 95) -> (-95, -95)
  line L7 (0, 85) -> (0, -85) construction
  line L8 (-85, 85) -> (-85, -85)
  line L9 (95, 95) -> (-95, -95) construction
  line L10 (95, -95) -> (95, 95)
  line L11 (90, 90) -> (-90, 90)
  line L12 (-90, -90) -> (90, -90)
  line L13 (-85, 0) -> (85, 0) construction
  line L14 (-95, -95) -> (95, -95)
  line L15 (-90, 90) -> (-90, -90)
  dimension "d3" = -5
  dimension "d4" = -5
  dimension "d5" = 190
  dimension "d6" = 190
  constraint horizontal L2
  constraint perpendicular L2 L6
  constraint parallel L2 L14
  constraint parallel L6 L10
  constraint coincident origin L9
  constraint coincident origin L1
  constraint midpoint L13.start L8
  constraint midpoint L13.end L5
  constraint midpoint L7.start L3
  constraint midpoint L7.end L4
  measures "d5" distance of L6.end L1.end
  measures "d6" distance of L1.start L6.end
extrude "Extrude4" add sketch "Sketch1" along normal mid plane 50 contours L0 L11 L12 L15
extrude "Extrude5" add sketch "Sketch1" along normal mid plane 60 contours L2 L6 L10 L14
sketch "Sketch2" plane through (0, 0, -85) normal (0, 0, 1) x (-1, 0, 0)
  line L0 (25, 85) -> (-25, 85)
  line L1 (-25, 85) -> (-25, -85)
  line L2 (-25, -85) -> (25, -85)
  line L3 (25, -85) -> (25, 85)
  line L4 (-2.525, 85) -> (2.525, 85)
  line L5 (2.525, 85) -> (2.525, -85)
  line L6 (2.525, -85) -> (-2.525, -85)
  line L7 (-2.525, -85) -> (-2.525, 85)
  line L8 (-2.525, 85) -> (2.525, -85) construction
  line L9 (2.525, 85) -> (-2.525, -85) construction
  line L10 (5.025, 87.5) -> (5.025, -87.5)
  line L11 (5.025, -87.5) -> (-5.025, -87.5)
  line L12 (-5.025, -87.5) -> (-5.025, 87.5)
  line L13 (-5.025, 87.5) -> (5.025, 87.5)
  dimension "d39" = -2.5
  dimension "d40" = 5.05
  constraint horizontal L4
  constraint perpendicular L4 L5
  constraint parallel L4 L6
  constraint parallel L5 L7
  constraint coincident L8 origin
  constraint coincident L9 origin
  constraint coincident L0 L4.start
  measures "d40" distance of L5 L7
extrude "Extrude6" add sketch "Sketch2" along normal blind 5 contours L0 L2 L5 L10 | L0 L2 L7 L12
sketch "Sketch3" plane through (0, 0, 85) normal (0, 0, -1) x (1, 0, 0)
  line L0 (-25, -85) -> (25, -85)
  line L1 (25, -85) -> (25, 85)
  line L2 (25, 85) -> (-25, 85)
  line L3 (-25, 85) -> (-25, -85)
  line L4 (-2.5, 85) -> (2.5, 85)
  line L5 (2.5, 85) -> (2.5, -85)
  line L6 (2.5, -85) -> (-2.5, -85)
  line L7 (-2.5, -85) -> (-2.5, 85)
  line L8 (-2.5, 85) -> (2.5, -85) construction
  line L9 (2.5, 85) -> (-2.5, -85) construction
  line L10 (5, 87.5) -> (5, -87.5)
  line L11 (5, -87.5) -> (-5, -87.5)
  line L12 (-5, -87.5) -> (-5, 87.5)
  line L13 (-5, 87.5) -> (5, 87.5)
  dimension "d43" = 5
  dimension "d44" = -2.5
  constraint horizontal L4
  constraint perpendicular L4 L5
  constraint parallel L4 L6
  constraint parallel L5 L7
  constraint coincident L8 origin
  constraint coincident L9 origin
  measures "d43" distance of L5.end L6.end
extrude "Extrude7" add sketch "Sketch3" along normal blind 5 contours L0 L2 L7 L12 | L0 L2 L5 L10
equation "d6 = d5"
named bodies: "Cutie mijloc"
